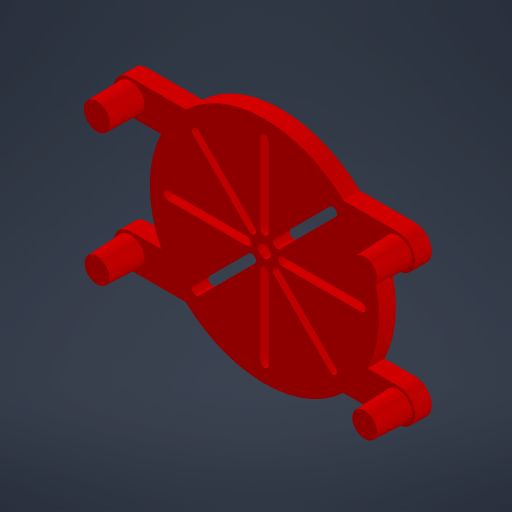
# Autodesk Inventor part: Laser Alignment Tool V2
Saved by Autodesk Inventor 2023.4 (Build 274418000, 418)
## iProperties
Created: 2022-11-15
Part Number: Laser Alignment Tool V2
Material: Generic
Document SubType Name: Modeling
Designer: xSibe
Density: 1 g/cm^3
Appearance: Plastic Dark Red
Author: xSibe
Autodesk Inventor part; units mm, degrees
ref_plane "YZ Plane" through (0, 0, 0) normal (1, 0, 0) x (0, 1, 0)
ref_plane "XZ Plane" through (0, 0, 0) normal (0, 1, 0) x (-1, 0, 0)
ref_plane "XY Plane" through (0, 0, 0) normal (0, 0, 1) x (1, 0, 0)
sketch "Sketch2" plane through (0, 0, 0) normal (0, 0, 1) x (0, 1, 0)
  line L0 (24.9, -57.75) -> (24.9, -91.85)
  circle A0 centre (24.9, -74.8) radius 17.05
  circle A1 centre (24.9, -74.8) radius 0.9375
  line L1 (24.9, -74.8) -> (36.9562, -86.8562)
  line L2 (24.9, -74.8) -> (41.95, -74.8) construction
  line L3 (26.7738, -76.6738) -> (35.0823, -84.9823) construction
  line L4 (26.3319, -77.1158) -> (34.6404, -85.4243)
  line L5 (35.5243, -84.5404) -> (27.2158, -76.2319)
  arc A2 (27.2158, -76.2319) -> (26.3319, -77.1158) centre (26.7738, -76.6738) ccw
  arc A3 (34.6404, -85.4243) -> (35.5243, -84.5404) centre (35.0823, -84.9823) ccw
  line L6 (30.9281, -80.8281) -> (42.6781, -80.8281) construction
  line L7 (34.8, -54.9) -> (34.8, -60.9186) construction
  line L8 (32.3, -54.9) -> (32.3, -60.9186)
  line L9 (37.3, -60.9186) -> (37.3, -54.9)
  arc A4 (37.3, -54.9) -> (32.3, -54.9) centre (34.8, -54.9) ccw
  arc A5 (32.3, -60.9186) -> (37.3, -60.9186) centre (34.8, -60.9186) ccw
  line L10 (15, -54.9) -> (15, -60.9186) construction
  line L11 (12.5, -54.9) -> (12.5, -60.9186)
  line L12 (17.5, -60.9186) -> (17.5, -54.9)
  arc A6 (17.5, -54.9) -> (12.5, -54.9) centre (15, -54.9) ccw
  arc A7 (12.5, -60.9186) -> (17.5, -60.9186) centre (15, -60.9186) ccw
  line L13 (15, -94.7) -> (15, -88.6814) construction
  line L14 (17.5, -94.7) -> (17.5, -88.6814)
  line L15 (12.5, -88.6814) -> (12.5, -94.7)
  arc A8 (12.5, -94.7) -> (17.5, -94.7) centre (15, -94.7) ccw
  arc A9 (17.5, -88.6814) -> (12.5, -88.6814) centre (15, -88.6814) ccw
  line L16 (34.8, -94.7) -> (34.8, -88.6814) construction
  line L17 (37.3, -94.7) -> (37.3, -88.6814)
  line L18 (32.3, -88.6814) -> (32.3, -94.7)
  arc A10 (32.3, -94.7) -> (37.3, -94.7) centre (34.8, -94.7) ccw
  arc A11 (37.3, -88.6814) -> (32.3, -88.6814) centre (34.8, -88.6814) ccw
  line L19 (39.3, -74.175) -> (27.55, -74.175)
  arc A12 (39.3, -75.425) -> (39.3, -74.175) centre (39.3, -74.8) ccw
  line L20 (27.55, -75.425) -> (39.3, -75.425)
  arc A13 (27.55, -74.175) -> (27.55, -75.425) centre (27.55, -74.8) ccw
  line L21 (34.6404, -64.1757) -> (26.3319, -72.4842)
  arc A14 (35.5243, -65.0596) -> (34.6404, -64.1757) centre (35.0823, -64.6177) ccw
  line L22 (27.2158, -73.3681) -> (35.5243, -65.0596)
  arc A15 (26.3319, -72.4842) -> (27.2158, -73.3681) centre (26.7738, -72.9262) ccw
  line L23 (24.275, -60.4) -> (24.275, -72.15)
  arc A16 (25.525, -60.4) -> (24.275, -60.4) centre (24.9, -60.4) ccw
  line L24 (25.525, -72.15) -> (25.525, -60.4)
  arc A17 (24.275, -72.15) -> (25.525, -72.15) centre (24.9, -72.15) ccw
  line L25 (14.2757, -65.0596) -> (22.5842, -73.3681)
  arc A18 (15.1596, -64.1757) -> (14.2757, -65.0596) centre (14.7177, -64.6177) ccw
  line L26 (23.4681, -72.4842) -> (15.1596, -64.1757)
  arc A19 (22.5842, -73.3681) -> (23.4681, -72.4842) centre (23.0262, -72.9262) ccw
  line L27 (10.5, -75.425) -> (22.25, -75.425)
  arc A20 (10.5, -74.175) -> (10.5, -75.425) centre (10.5, -74.8) ccw
  line L28 (22.25, -74.175) -> (10.5, -74.175)
  arc A21 (22.25, -75.425) -> (22.25, -74.175) centre (22.25, -74.8) ccw
  line L29 (15.1596, -85.4243) -> (23.4681, -77.1158)
  arc A22 (14.2757, -84.5404) -> (15.1596, -85.4243) centre (14.7177, -84.9823) ccw
  line L30 (22.5842, -76.2319) -> (14.2757, -84.5404)
  arc A23 (23.4681, -77.1158) -> (22.5842, -76.2319) centre (23.0262, -76.6738) ccw
  line L31 (25.525, -89.2) -> (25.525, -77.45)
  arc A24 (24.275, -89.2) -> (25.525, -89.2) centre (24.9, -89.2) ccw
  line L32 (24.275, -77.45) -> (24.275, -89.2)
  arc A25 (25.525, -77.45) -> (24.275, -77.45) centre (24.9, -77.45) ccw
  line L33 (37.3, -60.9186) -> (37.3, -88.6814)
  line L34 (12.5, -88.6814) -> (12.5, -60.9186)
  line L35 (0.025, -97.7) -> (0.025, -51.9) projected
  line L36 (42.1, -97.7) -> (0.025, -97.7) projected
  line L37 (42.1, -97.7) -> (42.1, -91.85) projected
  line L38 (7.7, -91.85) -> (42.1, -91.85) projected
  line L39 (7.7, -57.75) -> (7.7, -91.85) projected
  line L40 (7.7, -57.75) -> (42.1, -57.75) projected
  line L41 (42.1, -57.75) -> (42.1, -51.9) projected
  line L42 (0.025, -51.9) -> (42.1, -51.9) projected
  circle A26 centre (34.8, -94.7) radius 2.0625 projected
  circle A27 centre (34.8, -54.9) radius 2.0625 projected
  circle A28 centre (15, -94.7) radius 2.0625 projected
  circle A29 centre (15, -54.9) radius 2.0625 projected
  point P0 (0, 0)
  point P1 (34.8, -57.9093)
  point P2 (15, -57.9093)
  point P3 (15, -91.6907)
  point P4 (34.8, -91.6907)
  point P5 (17.5, -59.4396)
  point P6 (13.0765, -62.5156)
  point P7 (13.0765, -87.0844)
  point P8 (17.5, -90.1604)
  point P9 (32.3, -90.1604)
  point P10 (36.7235, -87.0844)
  point P11 (36.7235, -62.5156)
  point P12 (32.3, -59.4396)
  point P13 (12.5, -63.0978)
  point P14 (12.5, -86.5022)
  point P15 (37.3, -86.5022)
  point P16 (37.3, -63.0978)
  dimension "d32" = 1.875
  dimension "d33" = 45
  dimension "d34" = 5.875
  dimension "d35" = 45
  dimension "d36" = 1.25
  dimension "d37" = 5
  dimension "d38" = 5
  dimension "d39" = 5
  dimension "d40" = 5
  dimension "d43" = 360
  constraints: 80 end point, 54 point on circle, 26 centre point, 20 tangent, 9 midpoint, 6 coincident, 6 parallel, 3 vertical, 2 equal length, 2 horizontal, 2 point on line, 1 collinear, 81 other
  measures "d32" diameter of A1
  measures "d33" angle of L1 L2
  measures "d34" distance of L6.start L3.end
  measures "d35" angle of L3 L6
  measures "d36" diameter of A3
  measures "d37" diameter of A5
  measures "d38" diameter of A7
  measures "d39" diameter of A9
  measures "d40" diameter of A11
extrude "Extrusion2" add sketch "Sketch2" along normal mid plane 2.5 contours A0 L8 A5 L33 L19 A13 L20 L1 A3 L5 A2 A1 L0 A17 L24 A16 | L0 A16 L23 A17 A1 A25 L32 A24 A0 L14 A9 L34 L27 A21 L28 A7 L12 | L8 L40 L9 A5 A0 | A0 A5 L8 | L12 A7 A0 | A0 A7 L11 L40 L12 | L40 L11 A6 L12 | L8 A4 L9 L40 | A5 L33 A0 | A0 L34 A7 | A0 L33 L20 A12 L19 | L34 L28 A20 L27 A0 | A1 L1 A2 L4 A3 A0 A11 L18 L0 A24 L31 A25 | A0 A9 L34 | L33 A11 A0 | A9 L14 A0 | A0 L14 L38 L15 A9 | L38 L14 A8 L15 | L17 L38 L18 A0 A11 | A0 L18 A11 | L17 A10 L18 L38 | A26 | A27 | A28 | A29
sketch "Sketch3" plane through (0, 0, 1.25) normal (0, 0, 1) x (1, 0, 0)
  line L0 (97.7, 0.025) -> (51.9, 0.025) projected
  line L1 (97.7, 42.1) -> (97.7, 0.025) projected
  line L2 (97.7, 42.1) -> (91.85, 42.1) projected
  line L3 (91.85, 7.7) -> (91.85, 42.1) projected
  line L4 (57.75, 7.7) -> (91.85, 7.7) projected
  line L5 (57.75, 7.7) -> (57.75, 42.1) projected
  line L6 (57.75, 42.1) -> (51.9, 42.1) projected
  line L7 (51.9, 0.025) -> (51.9, 42.1) projected
  circle A0 centre (94.7, 34.8) radius 2.0625 projected
  circle A1 centre (54.9, 34.8) radius 2.0625 projected
  circle A2 centre (94.7, 15) radius 2.0625 projected
  circle A3 centre (54.9, 15) radius 2.0625 projected
  point P0 (0, 0)
extrude "Extrusion3" add sketch "Sketch3" along normal blind 5 contours A0 | A1 | A2 | A3
chamfer "Chamfer1" distance 5 angle 1 1 edges at (52.8375, 34.8, 6.25) measured on face at (52.8642, 35.1308, 2.9167)
chamfer "Chamfer2" distance 5 angle 2.5 1 edges at (92.6375, 34.8, 6.25) measured on face at (95.5842, 36.6634, 4.5833)
chamfer "Chamfer3" distance 5 angle 2.5 1 edges at (52.8375, 15, 6.25) measured on face at (56.9358, 14.6692, 4.5833)
chamfer "Chamfer4" distance 5 angle 2.5 1 edges at (92.6375, 15, 6.25) measured on face at (93.8158, 13.1366, 4.5833)
body "Solid1"
